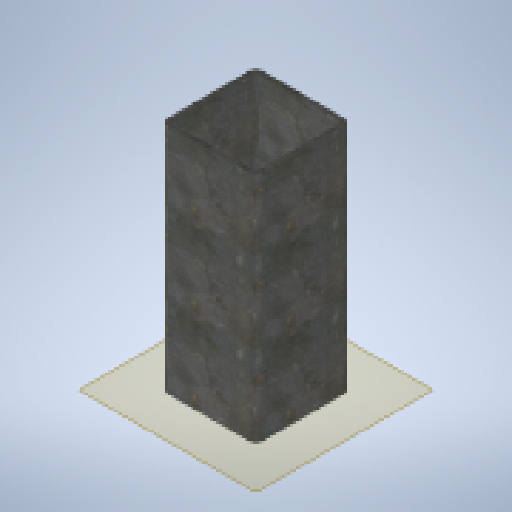
# Autodesk Inventor part: Central
Saved by Autodesk Inventor 2025.2 (Build 292293000, 293)
## iProperties
Created: 2025-04-01
Part Number: Central
Material: Steel
Document SubType Name: Modeling
Designer: bless
Density: 7.85 g/cm^3
Appearance: Plate
Author: bless
Autodesk Inventor part; units mm, degrees
ref_plane "YZ Plane" through (0, 0, 0) normal (1, 0, 0) x (0, 1, 0)
ref_plane "XZ Plane" through (0, 0, 0) normal (0, 1, 0) x (-1, 0, 0)
ref_plane "XY Plane" through (0, 0, 0) normal (0, 0, 1) x (1, 0, 0)
ref_plane "Work Plane1" through (90.3084, 93.6473, -291.2729) normal (0, 1, 0) x (-1, 0, 0)
sketch "Sketch1" plane through (90.3084, 93.6473, -291.2729) normal (0, 1, 0) x (-1, 0, 0)
  line L0 (87.5, 102.5) -> (-87.5, 102.5)
  line L1 (-102.5, 87.5) -> (-102.5, -87.5)
  line L2 (-87.5, -102.5) -> (87.5, -102.5)
  line L3 (102.5, -87.5) -> (102.5, 87.5)
  line L4 (102.5, 102.5) -> (-102.5, -102.5) construction
  line L5 (-102.5, 102.5) -> (102.5, -102.5) construction
  line L6 (87.5, 92.5) -> (-87.5, 92.5)
  line L7 (-92.5, 87.5) -> (-92.5, -87.5)
  line L8 (-87.5, -92.5) -> (87.5, -92.5)
  line L9 (92.5, -87.5) -> (92.5, 87.5)
  line L10 (92.5, 92.5) -> (-92.5, -92.5) construction
  line L11 (-92.5, 92.5) -> (92.5, -92.5) construction
  arc A0 (102.5, 87.5) -> (87.5, 102.5) centre (87.5, 87.5) ccw
  arc A1 (-87.5, 102.5) -> (-102.5, 87.5) centre (-87.5, 87.5) ccw
  arc A2 (-102.5, -87.5) -> (-87.5, -102.5) centre (-87.5, -87.5) ccw
  arc A3 (87.5, -102.5) -> (102.5, -87.5) centre (87.5, -87.5) ccw
  arc A4 (92.5, 87.5) -> (87.5, 92.5) centre (87.5, 87.5) ccw
  arc A5 (87.5, -92.5) -> (92.5, -87.5) centre (87.5, -87.5) ccw
  arc A6 (-92.5, -87.5) -> (-87.5, -92.5) centre (-87.5, -87.5) ccw
  arc A7 (-87.5, 92.5) -> (-92.5, 87.5) centre (-87.5, 87.5) ccw
  arc A8 (25, -173.2051) -> (173.2051, -25) centre (0, 0) ccw projected
  line L12 (25, -135) -> (25, -173.2051) projected
  point P0 (90.3084, 291.2729)
  dimension "d0" = 205
  dimension "d1" = 205
  dimension "d2" = 10
  dimension "d3" = 15
  dimension "d4" = 5
  constraints: 24 end point, 17 point on line, 16 point on circle, 16 tangent, 8 centre point, 6 equal radius, 4 midpoint, 4 parallel, 2 coincident, 2 horizontal, 2 perpendicular
  measures "d0" distance of L5.end L4.end
  measures "d1" distance of L4.end L5.start
  measures "d2" distance between parallel lines of L9 L3
  measures "d3" radius of A0
  measures "d4" radius of A4
extrude "Extrusion1" add sketch "Sketch1" along normal blind 500
body "Solid1"
